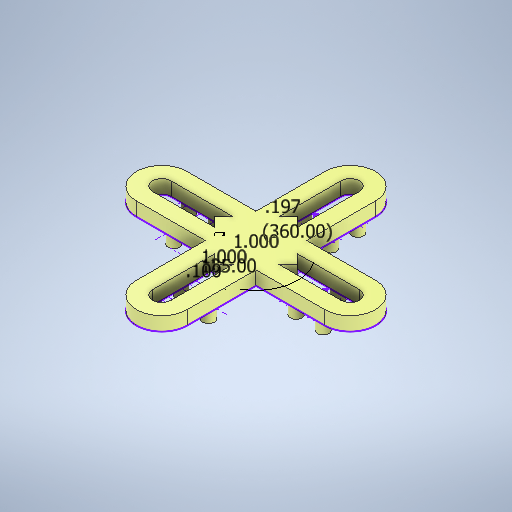
# Autodesk Inventor part: Redesign_Gripper_Baseplate
Saved by Autodesk Inventor 2025.1 (Build 291241000, 241)
## iProperties
Created: 2024-12-19
Part Number: Redesign_Gripper_Baseplate
Material: Generic
Document SubType Name: Modeling
Designer: m_kni
Density: 1 g/cm^3
Appearance: Default
Author: m_kni
Autodesk Inventor part; units mm, degrees
ref_plane "YZ Plane" through (0, 0, 0) normal (1, 0, 0) x (0, 1, 0)
ref_plane "XZ Plane" through (0, 0, 0) normal (0, 1, 0) x (-1, 0, 0)
ref_plane "XY Plane" through (0, 0, 0) normal (0, 0, 1) x (1, 0, 0)
sketch "Sketch1" plane through (0, 0, 0) normal (0, 1, 0) x (-1, 0, 0)
  line L0 (17.9605, 0) -> (0, -17.9605)
  line L1 (17.9605, 0) -> (43.3605, 0) construction
  line L2 (17.9605, 0) -> (0, 17.9605)
  line L3 (17.9605, 0) -> (43.3605, 0) construction
  line L4 (-17.9605, 0) -> (0, -17.9605)
  line L5 (-17.9605, 0) -> (0, 17.9605)
  line L6 (0, 15.4205) -> (-15.4205, 0)
  line L7 (0, 15.4205) -> (21.8079, 15.4205) construction
  line L8 (-15.4205, 0) -> (0, -15.4205)
  line L9 (0, -15.4205) -> (15.4205, 0)
  line L10 (15.4205, 0) -> (0, 15.4205)
  line L11 (0, -40.8205) -> (2, -40.8205)
  line L12 (0, -40.8205) -> (-2, -40.8205)
  circle A0 centre (7.5, -28.1205) radius 2.5
  line L13 (4, -28.1205) -> (4, -13.9605)
  line L14 (4, -28.1205) -> (4, -40.8205)
  line L15 (11, -6.9605) -> (11, -40.8205)
  arc A1 (-4, -40.8205) -> (4, -40.8205) centre (0, -40.8205) ccw
  line L16 (0, -15.4205) -> (0, -17.9605)
  line L17 (-4, -40.8205) -> (-4, -13.9605)
  line L18 (-11, -40.8205) -> (-11, -6.9605)
  arc A2 (-11, -40.8205) -> (11, -40.8205) centre (0, -40.8205) ccw
  circle A3 centre (-7.5, -24.8705) radius 2.5
  circle A4 centre (-7.5, -36.6205) radius 2.5
  line L19 (15.4205, 0) -> (17.9605, 0)
  line L20 (28.1205, 4) -> (13.9605, 4)
  circle A5 centre (28.1205, 7.5) radius 2.5
  circle A6 centre (24.8705, -7.5) radius 2.5
  line L21 (6.9605, 11) -> (40.8205, 11)
  line L22 (40.8205, -11) -> (6.9605, -11)
  line L23 (40.8205, -4) -> (13.9605, -4)
  line L24 (28.1205, 4) -> (40.8205, 4)
  line L25 (40.8205, 0) -> (40.8205, 2)
  circle A7 centre (36.6205, -7.5) radius 2.5
  line L26 (40.8205, 0) -> (40.8205, -2)
  arc A8 (40.8205, -4) -> (40.8205, 4) centre (40.8205, 0) ccw
  arc A9 (40.8205, -11) -> (40.8205, 11) centre (40.8205, 0) ccw
  line L27 (0, 15.4205) -> (0, 17.9605)
  line L28 (-4, 28.1205) -> (-4, 13.9605)
  circle A10 centre (-7.5, 28.1205) radius 2.5
  circle A11 centre (7.5, 24.8705) radius 2.5
  line L29 (-11, 6.9605) -> (-11, 40.8205)
  line L30 (11, 40.8205) -> (11, 6.9605)
  line L31 (4, 40.8205) -> (4, 13.9605)
  line L32 (-4, 28.1205) -> (-4, 40.8205)
  line L33 (0, 40.8205) -> (-2, 40.8205)
  circle A12 centre (7.5, 36.6205) radius 2.5
  line L34 (0, 40.8205) -> (2, 40.8205)
  arc A13 (4, 40.8205) -> (-4, 40.8205) centre (0, 40.8205) ccw
  arc A14 (11, 40.8205) -> (-11, 40.8205) centre (0, 40.8205) ccw
  line L35 (-15.4205, 0) -> (-17.9605, 0)
  line L36 (-28.1205, -4) -> (-13.9605, -4)
  circle A15 centre (-28.1205, -7.5) radius 2.5
  circle A16 centre (-24.8705, 7.5) radius 2.5
  line L37 (-6.9605, -11) -> (-40.8205, -11)
  line L38 (-40.8205, 11) -> (-6.9605, 11)
  line L39 (-40.8205, 4) -> (-13.9605, 4)
  line L40 (-28.1205, -4) -> (-40.8205, -4)
  line L41 (-40.8205, 0) -> (-40.8205, -2)
  circle A17 centre (-36.6205, 7.5) radius 2.5
  line L42 (-40.8205, 0) -> (-40.8205, 2)
  arc A18 (-40.8205, 4) -> (-40.8205, -4) centre (-40.8205, 0) ccw
  arc A19 (-40.8205, 11) -> (-40.8205, -11) centre (-40.8205, 0) ccw
  point P0 (0, 0)
  point P1 (0, -28.1205)
  point P2 (2, -28.1205)
  point P3 (-2, -22.1205)
  point P4 (-7.5, -22.1205)
  point P5 (-2, -34.1205)
  point P6 (-7.5, -34.1205)
  point P7 (11, -28.1205)
  point P8 (28.1205, 2)
  point P9 (28.1205, 11)
  point P10 (34.1205, -7.5)
  point P11 (34.1205, -2)
  point P12 (22.1205, -7.5)
  point P13 (22.1205, -2)
  point P14 (28.1205, 0)
  point P15 (-2, 28.1205)
  point P16 (-11, 28.1205)
  point P17 (7.5, 34.1205)
  point P18 (2, 34.1205)
  point P19 (7.5, 22.1205)
  point P20 (2, 22.1205)
  point P21 (0, 28.1205)
  point P22 (-28.1205, -2)
  point P23 (-28.1205, -11)
  point P24 (-34.1205, 7.5)
  point P25 (-34.1205, 2)
  point P26 (-22.1205, 7.5)
  point P27 (-22.1205, 2)
  point P28 (-28.1205, 0)
  point P29 (11, 11)
  point P30 (-11, 11)
  point P31 (-11, -11)
  point P32 (11, -11)
  dimension "d12" = 25.4
  dimension "d15" = 25.4
  dimension "d18" = 2.54
  dimension "d19" = 135
  dimension "d25" = 5
  dimension "d41" = 360
  constraints: 86 end point, 20 centre point, 16 coincident, 16 point on circle, 12 point on line, 5 vertical, 4 parallel, 3 equal length, 3 horizontal, 3 perpendicular, 173 other
  measures "d12" distance of L0.start L0.end
  measures "d15" distance of L0.start L2.end
  measures "d18" distance of L6.start L2.end
  measures "d19" angle of L6 L7
  measures "d25" diameter of A0
extrude "Extrusion1" add sketch "Sketch1" along normal blind 6 contours L19 L10 L27 L2 | L0 L16 L9 L19 | L23 A8 L24 L20 L2 L30 L21 A9 L22 L15 L0 | L9 L8 L6 L10 | L15 L22 L0 | L2 L21 L30 | L16 L4 L35 L8 | L6 L35 L5 L27 | L22 L15 A2 L18 L37 L4 L17 A1 L14 L13 L0 | L2 L31 A13 L32 L28 L5 L38 L29 A14 L30 L21 | L4 L18 L37 A19 L38 L29 L5 L39 A18 L40 L36 | L37 L18 L4 | L5 L29 L38 | A0 | A3 | A4 | A5 | A6 | A7 | A10 | A11 | A12 | A15 | A16 | A17
extrude "Extrusion2" add sketch "Sketch1" against normal blind 5.6 contours A0 | A3 | A4 | A5 | A6 | A7 | A10 | A11 | A12 | A15 | A16 | A17
sketch "Sketch2" plane through (0, 0, 0) normal (0, -1, 0) x (1, 0, 0)
  circle A0 centre (7.5, 28.1205) radius 2.5 projected
  circle A1 centre (7.5, 28.1205) radius 2.625
  circle A2 centre (-7.5, 36.6205) radius 2.5 projected
  circle A3 centre (-7.5, 36.6205) radius 2.625
  circle A4 centre (-7.5, 24.8705) radius 2.5 projected
  circle A5 centre (-7.5, 24.8705) radius 2.625
  circle A6 centre (-28.1205, 7.5) radius 2.625
  circle A7 centre (-36.6205, -7.5) radius 2.625
  circle A8 centre (-24.8705, -7.5) radius 2.625
  circle A9 centre (-7.5, -28.1205) radius 2.625
  circle A10 centre (7.5, -36.6205) radius 2.625
  circle A11 centre (7.5, -24.8705) radius 2.625
  circle A12 centre (28.1205, -7.5) radius 2.625
  circle A13 centre (36.6205, 7.5) radius 2.625
  circle A14 centre (24.8705, 7.5) radius 2.625
  point P0 (0, 0)
  dimension "d47" = 5.25
  dimension "d48" = 5.25
  dimension "d49" = 5.25
  dimension "d52" = 360
  constraints: 12 centre point, 3 coincident, 25 other
  measures "d47" diameter of A1
  measures "d48" diameter of A3
  measures "d49" diameter of A5
extrude "Extrusion3" add sketch "Sketch2" along normal blind 0.6 contours A0 | A1 | A2 | A3 | A4 | A5 | A6 | A7 | A8 | A9 | A10 | A11 | A12 | A13 | A14
sketch "Sketch3" plane through (7.5, -5.6, 28.1205) normal (0, -1, 0) x (1, 0, 0)
  circle A0 centre (0, 0) radius 2
  circle A1 centre (-15, 8.5) radius 2.5 projected
  circle A2 centre (-15, 8.5) radius 2
  circle A3 centre (-15, -3.25) radius 2.5 projected
  circle A4 centre (-15, -3.25) radius 2
  circle A5 centre (-44.1205, -35.6205) radius 2
  circle A6 centre (-32.3705, -35.6205) radius 2
  circle A7 centre (-35.6205, -20.6205) radius 2
  circle A8 centre (0, -64.741) radius 2
  circle A9 centre (0, -52.991) radius 2
  circle A10 centre (-15, -56.241) radius 2
  circle A11 centre (29.1205, -20.6205) radius 2
  circle A12 centre (17.3705, -20.6205) radius 2
  circle A13 centre (20.6205, -35.6205) radius 2
  point P0 (-7.5, -28.1205)
  dimension "d56" = 4
  dimension "d57" = 4
  dimension "d58" = 4
  dimension "d61" = 360
  constraints: 12 centre point, 2 coincident, 25 other
  measures "d56" diameter of A0
  measures "d57" diameter of A2
  measures "d58" diameter of A4
extrude "Extrusion4" cut sketch "Sketch3" against normal blind 6 contours A0 | A2 | A4 | A5 | A6 | A7 | A8 | A9 | A10 | A11 | A12 | A13
body "Solid1"
